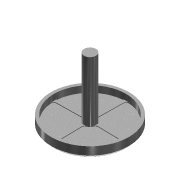
# Autodesk Inventor part: 上导轨
Saved by Autodesk Inventor 2021 (Build 250183000, 183)
## iProperties
Created: 2024-06-10
Part Number: 上导轨
Material: 常规
Document SubType Name: Modeling
Designer: 86155
Density: 1 g/cm^3
Appearance: 默认
Author: 86155
Autodesk Inventor part; units mm, degrees
ref_plane "YZ Plane" through (0, 0, 0) normal (1, 0, 0) x (0, 1, 0)
ref_plane "XZ Plane" through (0, 0, 0) normal (0, 1, 0) x (-1, 0, 0)
ref_plane "XY Plane" through (0, 0, 0) normal (0, 0, 1) x (1, 0, 0)
sketch "草图1" plane through (0, 0, 0) normal (0, 1, 0) x (-1, 0, 0)
  circle A0 centre (0, 0) radius 650
  dimension "d0" = 1300
  constraints: 1 centre point, 1 coincident
  measures "d0" diameter of A0
extrude "拉伸1" add sketch "草图1" along normal blind 30
sketch "草图2" plane through (0, 0, 0) normal (1, 0, 0) x (0, 1, 0)
  line L0 (0, 570) -> (-30, 570)
  line L1 (-30, 570) -> (-30, 600)
  line L2 (-30, 600) -> (0, 600)
  line L3 (0, 600) -> (0, 570)
  line L4 (0, -650) -> (0, 650) projected
  point P0 (0, 0)
  dimension "d3" = 30
  dimension "d4" = 30
  dimension "d7" = 50
  constraints: 8 end point, 2 parallel, 1 horizontal, 1 perpendicular
  measures "d3" distance between parallel lines of L0 L2
  measures "d4" distance between parallel lines of L3 L1
  measures "d7" distance of L4.end L2.end
sketch "草图3" plane through (0, 0, 0) normal (0, -1, 0) x (1, 0, 0)
  circle A0 centre (0, 0) radius 600
  dimension "d8" = 1200
  constraints: 1 centre point, 1 coincident
  measures "d8" diameter of A0
sweep "扫掠1" add profiles "草图2" path "草图3"
sketch "草图4" plane through (0, 0, 0) normal (0, 0, 1) x (1, 0, 0)
  line L0 (-600, -30) -> (600, -30) projected
  line L1 (-570, -30) -> (570, -30) projected
  line L2 (600, -30) -> (570, -30)
  line L3 (575, -60) -> (595, -60)
  line L4 (570, -55) -> (570, -50)
  line L5 (570, -30) -> (570, -40)
  arc A0 (570, -50) -> (570, -40) centre (570, -45) ccw
  arc A1 (600, -40) -> (600, -50) centre (600, -45) ccw
  line L6 (600, -55) -> (600, -50)
  line L7 (600, -40) -> (600, -30)
  line L8 (575, -60) -> (570, -55)
  line L9 (595, -60) -> (600, -55)
  point P0 (0, 0)
  point P1 (570, -60)
  point P2 (600, -60)
  dimension "d12" = 10
  dimension "d13" = 10
  dimension "d14" = 5
  dimension "d15" = 5
  dimension "d16" = 5
  dimension "d17" = 5
  dimension "d18" = 5
  constraints: 16 end point, 4 point on circle, 4 point on line, 2 centre point, 1 horizontal, 1 parallel, 1 perpendicular, 1 vertical
  measures "d12" distance of point (570, -60) L4.end
  measures "d13" distance of L2.end L5.end
  measures "d14" radius of A0
  measures "d15" distance of L3.start point (570, -60)
  measures "d16" distance of L4.start point (570, -60)
  measures "d17" distance of L3.end point (600, -60)
  measures "d18" distance of L6.start point (600, -60)
sketch3d "三维草图1"
  arc A0 (570, -30, 0) -> (0, -30, 570) centre (0, -30, 0) ccw
  arc A1 (0, -30, 570) -> (-570, -30, 0) centre (0, -30, 0) ccw
  arc A2 (-570, -30, 0) -> (0, -30, -570) centre (0, -30, 0) ccw
  arc A3 (0, -30, -570) -> (570, -30, 0) centre (0, -30, 0) ccw
sweep "扫掠2" add profiles "草图4" path "三维草图1"
sketch "草图6" plane through (0, 30, 0) normal (0, 1, 0) x (1, 0, 0)
  circle A0 centre (0, 0) radius 650
  circle A1 centre (0, 0) radius 650 projected
  circle A2 centre (0, 0) radius 600
  constraints: 2 centre point, 2 coincident
extrude "拉伸3" add sketch "草图6" along normal blind 100
sketch "草图7" plane through (0, 30, 0) normal (0, 1, 0) x (1, 0, 0)
  circle A0 centre (0, 0) radius 100
  dimension "d35" = 200
  constraints: 1 centre point, 1 coincident
  measures "d35" diameter of A0
extrude "拉伸4" add sketch "草图7" along normal blind 1000
sketch "草图8" plane through (0, 0, 0) normal (0, -1, 0) x (1, 0, 0)
  circle A0 centre (0, 0) radius 15
  dimension "d38" = 30
  constraints: 1 centre point, 1 coincident
  measures "d38" diameter of A0
sketch "草图9" plane through (0, 0, 0) normal (0, -1, 0) x (1, 0, 0)
  point P0 (0, 0)
extrude "拉伸5" cut sketch "草图8" against normal blind 50
scale "缩放比例1" factors (0.4, 0.4, 0.4) then translate (0, 0, 0) bodies 1
sketch "草图10" plane through (0, 12, 0) normal (0, 1, 0) x (1, 0, 0)
  circle A0 centre (0, 0) radius 6 projected
  line L0 (0, 0) -> (240, 0)
  circle A1 centre (0, 0) radius 240 projected
  line L1 (0, 0) -> (74.1641, 228.2536)
  line L2 (0, 0) -> (-194.1641, 141.0685)
  line L3 (0, 0) -> (-194.1641, -141.0685)
  line L4 (0, 0) -> (74.1641, -228.2536)
  circle A2 centre (0, 0) radius 50
  line L5 (0, -5) -> (240, -5)
  line L6 (0, 5) -> (240, 5)
  point P0 (239.9479, 5)
  point P1 (49.7494, 5)
  point P2 (49.7494, -5)
  point P3 (239.9479, -5)
  dimension "d46" = 360
  dimension "d48" = 100
  dimension "d49" = 5
  dimension "d50" = 5
  constraints: 14 end point, 2 parallel, 1 centre point, 1 coincident, 1 horizontal, 18 other
  measures "d48" diameter of A2
  measures "d49" distance between parallel lines of L0 L5
  measures "d50" distance between parallel lines of L0 L6
extrude "拉伸6" add sketch "草图10" along normal blind 30 contours A2 L6 A1 L0 | L0 A1 L5 A2
pattern_circular "环形阵列2" count 5 over 360 about axis through (0, 12, 0) along (0, 1, 0) of "拉伸6"
extrude "拉伸7" add sketch "草图10" along normal blind 40 contours L0 A2 L5 A0 | A0 L6 A2 L0 | A0 L1 A2 L6 | L5 A2 L4 A0 | A0 L2 A2 L1 | L4 A2 L3 A0 | A0 L3 A2 L2
equation "\"d16\" = d15"
equation "\"d17\" = d15"
equation "\"d18\" = d17"
